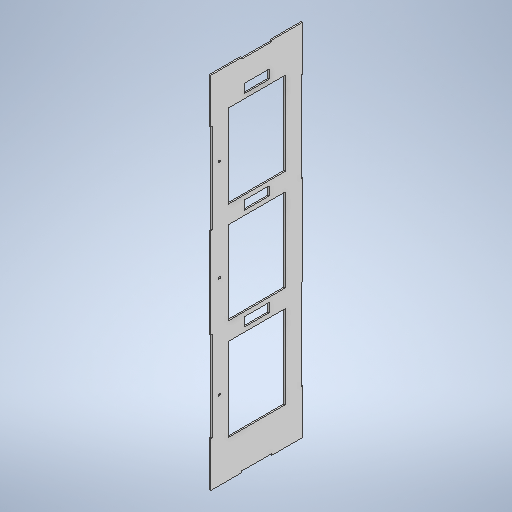
# Autodesk Inventor part: PAREDE FRONTAL
Saved by Autodesk Inventor 2025.2 (Build 292293000, 293)
## iProperties
Created: 2025-05-08
Part Number: PAREDE FRONTAL
Material: Genérico
Document SubType Name: Modeling
Designer: erick
Density: 1 g/cm^3
Appearance: Padrão
Author: erick
Autodesk Inventor part; units mm, degrees
ref_plane "YZ Plane" through (0, 0, 0) normal (1, 0, 0) x (0, 1, 0)
ref_plane "XZ Plane" through (0, 0, 0) normal (0, 1, 0) x (-1, 0, 0)
ref_plane "XY Plane" through (0, 0, 0) normal (0, 0, 1) x (1, 0, 0)
sketch "Esboço1" plane through (0, 0, 0) normal (1, 0, 0) x (0, 1, 0)
  line L0 (-504, 129) -> (504, 129)
  line L1 (504, 129) -> (504, -129)
  line L2 (504, -129) -> (-504, -129)
  line L3 (-504, -129) -> (-504, 129)
  line L4 (-504, 129) -> (504, -129) construction
  line L5 (504, 129) -> (-504, -129) construction
  point P0 (0, 0)
  dimension "d0" = 1008
  dimension "d1" = 258
  constraints: 12 end point, 2 midpoint, 2 parallel, 1 horizontal, 1 perpendicular
  measures "d0" distance of L1.end L2.end
  measures "d1" distance of L0.end L1.end
extrude "Extrusão1" add sketch "Esboço1" along normal mid plane 4
sketch "Esboço2" plane through (2, 0, 0) normal (1, 0, 0) x (0, 0, -1)
  line L0 (-133, 378) -> (-125, 378)
  line L1 (-125, 378) -> (-125, 126)
  line L2 (-125, 126) -> (-133, 126)
  line L3 (-133, 126) -> (-133, 378)
  line L4 (-129, 504) -> (-129, -504) projected
  line L5 (-133, 378) -> (-125, 126) construction
  line L6 (-125, 378) -> (-133, 126) construction
  line L7 (129, 504) -> (-129, 504) projected
  line L8 (-133, -126) -> (-125, -126)
  line L9 (-125, -126) -> (-125, -378)
  line L10 (-125, -378) -> (-133, -378)
  line L11 (-133, -378) -> (-133, -126)
  line L12 (-133, -126) -> (-125, -378) construction
  line L13 (-125, -126) -> (-133, -378) construction
  line L14 (-129, -504) -> (129, -504) projected
  line L15 (125, 378) -> (133, 378)
  line L16 (133, 378) -> (133, 126)
  line L17 (133, 126) -> (125, 126)
  line L18 (125, 126) -> (125, 378)
  line L19 (129, -504) -> (129, 504) projected
  line L20 (125, 378) -> (133, 126) construction
  line L21 (133, 378) -> (125, 126) construction
  line L22 (125, -126) -> (133, -126)
  line L23 (133, -126) -> (133, -378)
  line L24 (133, -378) -> (125, -378)
  line L25 (125, -378) -> (125, -126)
  line L26 (125, -126) -> (133, -378) construction
  line L27 (133, -126) -> (125, -378) construction
  point P0 (0, 0)
  point P1 (-129, 252)
  point P2 (-129, -252)
  point P3 (129, 252)
  point P4 (129, -252)
  dimension "d4" = 8
  dimension "d5" = 252
  dimension "d6" = 126
  dimension "d7" = 8
  dimension "d8" = 252
  dimension "d9" = 252
  dimension "d10" = 126
  dimension "d11" = 126
  dimension "d12" = 252
  dimension "d13" = 8
  dimension "d14" = 252
  dimension "d15" = 8
  dimension "d16" = 252
  dimension "d17" = 126
  constraints: 48 end point, 8 midpoint, 8 parallel, 4 horizontal, 4 perpendicular, 4 point on line
  measures "d4" distance of L0.start L0.end
  measures "d5" distance of L0.end L1.end
  measures "d6" distance between parallel lines of L0 L7
  measures "d7" distance of L9.end L10.end
  measures "d8" distance of L8.end L9.end
  measures "d9" distance between parallel lines of L8 L2
  measures "d10" distance between parallel lines of L14 L10
  measures "d11" distance between parallel lines of L15 L7
  measures "d12" distance of L15.end L16.end
  measures "d13" distance of L15.start L15.end
  measures "d14" distance between parallel lines of L22 L17
  measures "d15" distance of L22.start L22.end
  measures "d16" distance of L22.end L23.end
  measures "d17" distance between parallel lines of L14 L24
extrude "Extrusão2" cut sketch "Esboço2" along normal through all both and the other way through all contours L0 L4 L2 L3 | L0 L1 L2 L4 | L8 L9 L10 L4 | L4 L10 L11 L8 | L19 L17 L18 L15 | L15 L16 L17 L19 | L22 L23 L24 L19 | L19 L24 L25 L22
sketch "Esboço3" plane through (2, 0, 0) normal (1, 0, 0) x (0, 0, -1)
  line L0 (-41.5, 500) -> (41.5, 500)
  line L1 (41.5, 500) -> (41.5, 508)
  line L2 (41.5, 508) -> (-41.5, 508)
  line L3 (-41.5, 508) -> (-41.5, 500)
  line L4 (129, 504) -> (-129, 504) projected
  line L5 (-41.5, 500) -> (41.5, 508) construction
  line L6 (41.5, 500) -> (-41.5, 508) construction
  line L7 (-41.5, -500) -> (41.5, -500)
  line L8 (41.5, -500) -> (41.5, -508)
  line L9 (41.5, -508) -> (-41.5, -508)
  line L10 (-41.5, -508) -> (-41.5, -500)
  line L11 (-129, -504) -> (129, -504) projected
  line L12 (-41.5, -500) -> (41.5, -508) construction
  line L13 (41.5, -500) -> (-41.5, -508) construction
  point P0 (0, 0)
  point P1 (0, 504)
  point P2 (0, -504)
  dimension "d20" = 83
  dimension "d21" = 8
  dimension "d22" = 83
  dimension "d23" = 8
  constraints: 24 end point, 6 midpoint, 4 parallel, 2 horizontal, 2 perpendicular
  measures "d20" distance of L1.end L2.end
  measures "d21" distance of L0.end L1.end
  measures "d22" distance of L7.start L7.end
  measures "d23" distance of L7.end L8.end
extrude "Extrusão3" cut sketch "Esboço3" along normal through all both and the other way through all
sketch "Esboço5" plane through (2, 0, 0) normal (1, 0, 0) x (0, 0, -1)
  line L0 (41.5, 500) -> (-41.5, 500) projected
  line L1 (0, 400) -> (-80, 400)
  line L2 (-125, 378) -> (-125, 126) projected
  line L3 (0, 400) -> (80, 400)
  line L4 (-80, 400) -> (-80, 166.6667)
  line L5 (-80, 166.6667) -> (80, 166.6667)
  line L6 (80, 166.6667) -> (80, 400)
  point P0 (0, 0)
  dimension "d39" = 80
  dimension "d40" = 80
  dimension "d41" = 233.3333
  dimension "d67" = 45
  constraints: 10 end point, 2 horizontal, 2 perpendicular, 1 parallel
  measures "d39" distance of L1.start L1.end
  measures "d40" distance of L1.start L3.end
  measures "d41" distance of L1.end L4.end
  measures "d67" distance between parallel lines of L2 L4
extrude "Extrusão5" cut sketch "Esboço5" against normal through all
pattern_linear "Padrão retangular2" count 3 spacing 283.3333 along (0, -1, 0) of "Extrusão5"
sketch "Esboço6" plane through (2, 0, 0) normal (1, 0, 0) x (0, 0, -1)
  line L0 (-80, -166.6667) -> (80, -166.6667) projected
  line L1 (80, -116.6667) -> (-80, -116.6667) projected
  line L2 (-80, -116.6667) -> (-30, -116.6667)
  line L3 (80, -116.6667) -> (30, -116.6667)
  line L4 (30, -116.6667) -> (-30, -116.6667)
  line L5 (-35, -129.1667) -> (35, -129.1667)
  line L6 (35, -129.1667) -> (35, -154.1667)
  line L7 (35, -154.1667) -> (-35, -154.1667)
  line L8 (-35, -129.1667) -> (-35, -154.1667)
  line L9 (-125, -126) -> (-125, -378) projected
  point P0 (0, 0)
  point P1 (-35, -141.6667)
  dimension "d51" = 25
  dimension "d68" = 90
  dimension "d69" = 12.5
  dimension "d70" = 70
  constraints: 14 end point, 2 perpendicular, 2 point on line, 1 collinear, 1 midpoint, 1 vertical
  measures "d51" distance of L5.end L6.end
  measures "d68" distance from line of L9 point (-35, -141.667)
  measures "d69" distance between parallel lines of L1 L5
  measures "d70" distance of L5.start L5.end
extrude "Extrusão6" cut sketch "Esboço6" against normal through all
pattern_linear "Padrão retangular3" count 3 spacing 283.3333 along (0, 1, 0) of "Extrusão6"
sketch "Esboço7" plane through (2, 0, 0) normal (1, 0, 0) x (0, 0, -1)
  line L0 (-80, -400) -> (-80, -166.6667) projected
  line L1 (-125, -126) -> (-125, -378) projected
  line L2 (-80, 166.6667) -> (-80, 400) projected
  line L3 (-107.5, 280.8333) -> (-102.5, 280.8333)
  line L4 (-102.5, 280.8333) -> (-102.5, 285.8333)
  line L5 (-102.5, 285.8333) -> (-107.5, 285.8333)
  line L6 (-107.5, 285.8333) -> (-107.5, 280.8333)
  line L7 (-107.5, 280.8333) -> (-102.5, 285.8333) construction
  line L8 (-102.5, 280.8333) -> (-107.5, 285.8333) construction
  point P0 (0, 0)
  dimension "d60" = 5
  dimension "d61" = 5
  constraints: 12 end point, 2 parallel, 1 horizontal, 1 perpendicular
  measures "d60" distance of L5.end L4.end
  measures "d61" distance of L5.end L3.start
extrude "Extrusão7" cut sketch "Esboço7" against normal through all
pattern_linear "Padrão retangular4" count 3 spacing 283.3333 along (0, -1, 0) of "Extrusão7"
